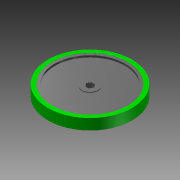
# Autodesk Inventor part: hjul
Saved by Autodesk Inventor 2012 (Build 160160000, 160)
## iProperties
Created: 2012-02-28
Part Number: hjul
Material: Default
Document SubType Name: Modeling
Designer: Grailas
Density: 1 g/cm^3
Author: Grailas
Autodesk Inventor part; units mm, degrees
ref_plane "YZ Plane" through (0, 0, 0) normal (1, 0, 0) x (0, 1, 0)
ref_plane "XZ Plane" through (0, 0, 0) normal (0, 1, 0) x (-1, 0, 0)
ref_plane "XY Plane" through (0, 0, 0) normal (0, 0, 1) x (1, 0, 0)
sketch "Sketch1" plane through (0, 0, 0) normal (0, 0, 1) x (1, 0, 0)
  circle A0 centre (0, 0) radius 71.375
  circle A1 centre (0, 0) radius 79.375
  line L0 (-3.6662, 6.35) -> (3.6662, 6.35)
  line L1 (3.6662, 6.35) -> (7.3323, 0)
  line L2 (7.3323, 0) -> (3.6662, -6.35)
  line L3 (3.6662, -6.35) -> (-3.6662, -6.35)
  line L4 (-3.6662, -6.35) -> (-7.3323, 0)
  line L5 (-7.3323, 0) -> (-3.6662, 6.35)
  circle A2 centre (0, 0) radius 66.375
  circle A3 centre (0, 0) radius 15.5
  point P0 (0, -6.35)
  dimension "d0" = 8
  dimension "d2" = 12.7
  dimension "d7" = 158.75
  dimension "d8" = 13
  dimension "d13" = 31
  constraints: 12 end point, 5 coincident, 4 centre point, 1 midpoint, 1 vertical alignment, 13 other
  measures "d0" radial gap between concentric circles of A0 A1
  measures "d2" distance between parallel lines of L0 L3
  measures "d7" diameter of A1
  measures "d8" radial gap between concentric circles of A2 A1
  measures "d13" diameter of A3
extrude "Extrusion1" add sketch "Sketch1" along normal mid plane 12.7 contours A0 | A1 | A2 | A3
extrude "Extrusion2" add sketch "Sketch1" along normal mid plane 20.32 contours A1
extrude "Extrusion3" add sketch "Sketch1" along normal blind 10 contours A0
extrude "Extrusion4" add sketch "Sketch1" against normal blind 10 contours A0
extrude "Extrusion5" add sketch "Sketch1" along normal mid plane 15.24 contours A3
body "Solid1"
